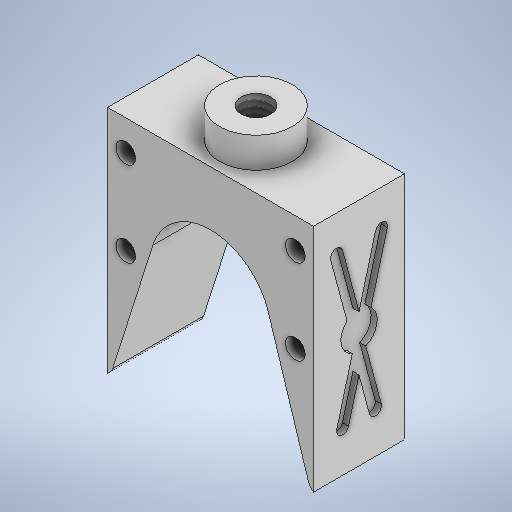
# Autodesk Inventor part: 2023
Saved by Autodesk Inventor 2025.1 (Build 291241000, 241)
## iProperties
Created: 2024-05-30
Part Number: 2023
Material: Generic
Document SubType Name: Modeling
Designer: Fabri
Density: 1 g/cm^3
Appearance: Default
Author: Fabri
Autodesk Inventor part; units mm, degrees
note: some values were not read from the file. Chosen so that the rebuilt part matches the saved one: direction of "Hole1"; direction of "Hole2".
ref_plane "XZ Plane" through (0, 0, 0) normal (0, 1, 0) x (-1, 0, 0)
ref_plane "XY Plane" through (0, 0, 0) normal (0, 0, 1) x (1, 0, 0)
sketch "Sketch1" plane through (0, 0, 0) normal (0, 1, 0) x (-1, 0, 0)
  line L0 (0, 0) -> (34, 0)
  line L1 (34, 0) -> (34, -38)
  line L2 (34, -38) -> (0, -38)
  line L3 (0, -38) -> (0, 0)
  point P0 (17, -38)
  dimension "d0" = 34
  dimension "d1" = 38
  constraints: 8 end point, 2 parallel, 1 horizontal, 1 midpoint, 1 perpendicular
  measures "d0" distance between parallel lines of L3 L1
  measures "d1" distance from line of point (17, -38) L0
extrude "Extrusion1" add sketch "Sketch1" along normal blind 15
sketch "Sketch2" plane through (0, 15, 0) normal (0, 1, 0) x (1, 0, 0)
  arc A0 (-26.5342, 15.9835) -> (-7.4658, 15.9835) centre (-17, 19) ccw
  line L0 (-26.5342, 15.9835) -> (-33.5, 38)
  line L1 (0, 38) -> (-34, 38) projected
  line L2 (-7.4658, 15.9835) -> (-0.5, 38)
  point P0 (0, 0)
  point P1 (-17, 38)
  dimension "d4" = 16.5
  dimension "d5" = 16.5
  dimension "d6" = 10
  dimension "d7" = 19
  constraints: 4 end point, 2 point on circle, 2 point on line, 2 tangent, 1 centre point, 1 midpoint, 1 vertical alignment
  measures "d4" horizontal distance of A0.centre L2.end
  measures "d5" horizontal distance of L0.end A0.centre
  measures "d6" radius of A0
  measures "d7" distance from line of L1 A0.centre
extrude "Extrusion2" cut sketch "Sketch2" against normal up to surface (15 mm away)
fillet "Fillet1" radius 2 2 edges at (-0.5, 7.5, -38) (-33.5, 7.5, -38)
sketch "Sketch3" plane through (0, 15, 0) normal (0, 1, 0) x (1, 0, 0)
  line L0 (-34, 0) -> (0, 0) projected
  point P0 (-3, 19)
  point P1 (-31, 19)
  point P2 (-17, 0)
  point P3 (-17, 0)
  point P4 (-34, 38)
  dimension "d19" = 14
  dimension "d20" = 14
  dimension "d59" = 19
  constraints: 2 midpoint, 1 horizontal alignment
  measures "d19" horizontal distance of point (-17, 0) point (-3, 19)
  measures "d20" horizontal distance of point (-17, 0) point (-31, 19)
  measures "d59" vertical distance of point (-34, 38) point (-31, 19)
hole "Hole1" at (-3, 15, -19) at (-31, 15, -19) direction (0, -1, 0) diameter 3.242 depth 15 thread size "M4x0.7" class "6H" standard "ISO Metric profile"
sketch "Sketch4" plane through (0, 15, 0) normal (0, 1, 0) x (1, 0, 0)
  line L0 (-34, 0) -> (0, 0) projected
  point P0 (-31, 5)
  point P1 (-3, 5)
  point P2 (-17, 0)
  point P3 (-17, 0)
  dimension "d28" = 14
  dimension "d29" = 14
  dimension "d30" = 5
  constraints: 2 midpoint, 1 horizontal alignment
  measures "d28" horizontal distance of point (-17, 0) point (-3, 5)
  measures "d29" horizontal distance of point (-17, 0) point (-31, 5)
  measures "d30" distance from line of L0 point (-3, 5)
hole "Hole2" at (-31, 15, -5) at (-3, 15, -5) direction (0, -1, 0) diameter 3.242 depth 15 thread size "M4x0.7" class "6H" standard "ISO Metric profile"
sketch "Sketch5" plane through (-34, 0, 0) normal (0, 0, 1) x (1, 0, 0)
  circle A0 centre (17, 7.5) radius 6
  line L0 (0, 0) -> (34, 0) projected
  line L1 (0, 0) -> (0, 15) projected
  point P0 (17, 0)
  point P1 (0, 7.5)
  dimension "d31" = 12
  constraints: 2 midpoint, 1 centre point, 1 horizontal alignment, 1 vertical alignment
  measures "d31" diameter of A0
extrude "Extrusion3" add sketch "Sketch5" along normal blind 5
sketch "Sketch6" plane through (-17, 7.5, 5) normal (0, 0, 1) x (1, 0, 0)
  circle A0 centre (0, 0) radius 6 projected
  point P0 (17, -7.5)
  constraints: 1 coincident
hole "Hole3" at (-17, 7.5, 5) direction (0, 0, -1) diameter 4.917 depth 15 thread size "M6x1" class "6H" standard "ISO Metric profile"
sketch "Sketch7" plane through (-34, 0, -38) normal (-1, 0, 0) x (0, 0, 1)
  line L0 (16.5986, 8.6063) -> (7.046, 11.1659)
  arc A0 (7.046, 11.1659) -> (6.5283, 9.2341) centre (6.7872, 10.2) ccw
  line L1 (6.5283, 9.2341) -> (13, 7.5)
  line L2 (13, 7.5) -> (6.5283, 5.7659)
  arc A1 (6.5283, 5.7659) -> (7.046, 3.8341) centre (6.7872, 4.8) ccw
  line L3 (7.046, 3.8341) -> (16.5986, 6.3937)
  line L4 (21.653, 9.4662) -> (31.7283, 12.1659)
  arc A2 (32.246, 10.2341) -> (31.7283, 12.1659) centre (31.9872, 11.2) ccw
  line L5 (32.246, 10.2341) -> (22.0423, 7.5)
  line L6 (22.0423, 7.5) -> (32.246, 4.7659)
  arc A3 (31.7283, 2.8341) -> (32.246, 4.7659) centre (31.9872, 3.8) ccw
  line L7 (31.7283, 2.8341) -> (21.653, 5.5338)
  line L8 (0, 0) -> (0, 15) projected
  line L9 (0, 7.5) -> (36.5337, 7.5) construction
  arc A4 (16.5986, 6.3937) -> (21.653, 5.5338) centre (19.3872, 7.5) ccw
  arc A5 (21.653, 9.4662) -> (16.5986, 8.6063) centre (19.3872, 7.5) ccw
  line L10 (0, 15) -> (38, 15) projected
  point P0 (38, 0)
  point P1 (11.8223, 5.1139)
  dimension "d42" = 2
  dimension "d43" = 2
  dimension "d44" = 2
  dimension "d45" = 2
  dimension "d46" = 12.6
  dimension "d47" = 12.6
  dimension "d48" = 26
  dimension "d49" = 26
  dimension "d50" = 30
  dimension "d51" = 30
  dimension "d52" = 3.8
  dimension "d53" = 3
  dimension "d54" = 3
  dimension "d55" = 13
  constraints: 18 end point, 12 point on circle, 8 tangent, 6 centre point, 4 parallel, 3 midpoint, 2 vertical alignment, 1 horizontal, 1 horizontal alignment, 1 point on line, 1 other
  measures "d42" distance from line of point (11.822, 5.114) L2
  measures "d43" distance between parallel lines of L1 L0
  measures "d44" distance between parallel lines of L5 L4
  measures "d45" distance between parallel lines of L7 L6
  measures "d46" horizontal distance of A3.centre A4.centre
  measures "d47" horizontal distance of A1.centre A4.centre
  measures "d48" distance of A2.centre A1.centre
  measures "d49" distance of A3.centre A0.centre
  measures "d50" angle of L6 L5
  measures "d51" angle of L2 L1
  measures "d52" distance from line of L10 A2.centre
  measures "d53" radius of A5
  measures "d54" radius of A4
  measures "d55" distance of point (0, 7.5) L1.end
extrude "Extrusion4" cut sketch "Sketch7" against normal blind 1
ref_plane "Work Plane1" through (-17, 0, 0) normal (1, 0, 0) x (0, 1, 0)
mirror "Mirror1" about plane through (-17, 0, 0) normal (1, 0, 0) of "Extrusion4"
equation "\"d5\" = d4"
equation "\"d20\" = d19"
equation "\"d12\" = d20"
equation "\"d29\" = d28"
equation "\"d42\" = d43"
equation "\"d44\" = d43"
equation "\"d47\" = d46"
equation "\"d54\" = d53"
body "Solid1"
